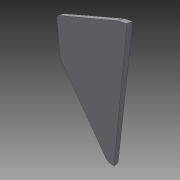
# Autodesk Inventor part: front_panel_brace_right
Saved by Autodesk Inventor 2014 (Build 180170000, 170)
## iProperties
Created: 2014-03-22
Part Number: front_panel_brace_right
Material: Generic
Document SubType Name: Modeling
Designer: buben
Density: 1 g/cm^3
Appearance: Default
Author: buben
Autodesk Inventor part; units mm, degrees
ref_plane "YZ Plane" through (0, 0, 0) normal (1, 0, 0) x (0, 1, 0)
ref_plane "XZ Plane" through (0, 0, 0) normal (0, 1, 0) x (-1, 0, 0)
ref_plane "XY Plane" through (0, 0, 0) normal (0, 0, 1) x (1, 0, 0)
sketch "Sketch1" plane through (0, 0, 0) normal (0, 1, 0) x (-1, 0, 0)
  line L0 (8, 0) -> (76.1537, -12.0173)
  line L1 (76.1537, -12.0173) -> (76.1537, -54.5039)
  line L2 (76.1537, -54.5039) -> (9.2866, -150)
  line L3 (0, -150) -> (0, 0)
  line L4 (75.1537, -50.7018) -> (69.8292, -46.9735) construction
  line L5 (69.8292, -46.9735) -> (1, -145.2718) construction
  line L6 (1, -145.2718) -> (6.3245, -149) construction
  line L7 (6.3245, -149) -> (75.1537, -50.7018) construction
  line L8 (75.1537, -14.8873) -> (74.0249, -21.2885) construction
  line L9 (74.0249, -21.2885) -> (1, -8.4123) construction
  line L10 (1, -8.4123) -> (2.1287, -2.011) construction
  line L11 (2.1287, -2.011) -> (75.1537, -14.8873) construction
  line L12 (73.1537, -45.9735) -> (66.6537, -45.9735) construction
  line L13 (66.6537, -45.9735) -> (66.6537, -22.2885) construction
  line L14 (66.6537, -22.2885) -> (73.1537, -22.2885) construction
  line L15 (73.1537, -22.2885) -> (73.1537, -45.9735) construction
  line L16 (0, -150) -> (9.2866, -150)
  line L17 (0, 0) -> (8, 0)
  line L18 (66.6537, -51.5086) -> (66.6537, -19.9888)
  point P0 (0, 0)
  dimension "d0" = 6.5
  dimension "d1" = 3
  dimension "d2" = 3
  dimension "d3" = 3
  dimension "d4" = 120
  dimension "d5" = 80
  dimension "d6" = 35
  dimension "d7" = 1
  dimension "d8" = 1
  dimension "d9" = 1
  dimension "d10" = 1
  dimension "d12" = 1
  dimension "d13" = 8
  dimension "d14" = 150
  constraints: 38 end point, 8 parallel, 7 perpendicular, 2 equal length, 2 point on line, 2 vertical alignment, 1 coincident, 1 collinear, 1 horizontal, 1 vertical
  measures "d0" distance of L12.start L12.end
  measures "d1" distance between parallel lines of L2 L7
  measures "d2" distance between parallel lines of L1 L15
  measures "d3" distance between parallel lines of L0 L11
  measures "d4" distance of L4.end L5.end
  measures "d5" angle of L3 L0
  measures "d6" angle of L3 L2
  measures "d7" distance from line of L9.end L3
  measures "d8" distance from line of L8.start L1
  measures "d9" distance from line of L4.end L12
  measures "d10" distance from line of L8.end L14
  measures "d12" distance from line of L6.end L16
  measures "d13" distance of L3.end L0.start
  measures "d14" distance of L3.start L3.end
extrude "Extrusion1" add sketch "Sketch1" along normal blind 6.5
chamfer "Chamfer1" distance 2 angle 45 3 edges at (-76.1537, 3.25, -54.5039) (-76.1537, 3.25, -12.0173) (-9.2866, 3.25, -150)
body "Solid1"
